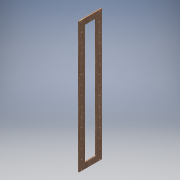
# Autodesk Inventor part: Arm
Saved by Autodesk Inventor 2019 (Build 230136000, 136)
## iProperties
Created: 2019-01-14
Part Number: Arm
Material: Wood (Birch)
Document SubType Name: Modeling
Designer: nxgam
Density: 0.55 g/cm^3
Appearance: Birch - Natural Polished
Author: nxgam
Autodesk Inventor part; units mm, degrees
ref_plane "YZ Plane" through (0, 0, 0) normal (1, 0, 0) x (0, 1, 0)
ref_plane "XZ Plane" through (0, 0, 0) normal (0, 1, 0) x (-1, 0, 0)
ref_plane "XY Plane" through (0, 0, 0) normal (0, 0, 1) x (1, 0, 0)
sketch "Sketch1" plane through (0, 0, 0) normal (1, 0, 0) x (0, 1, 0)
  line L0 (0, 50.8) -> (579.12, 50.8)
  line L1 (579.12, 50.8) -> (579.12, -50.8)
  line L2 (579.12, -50.8) -> (0, -50.8)
  line L3 (0, -50.8) -> (0, 50.8)
  point P0 (0, 0)
  point P1 (0, 0)
  dimension "d0" = 579.12
  dimension "d1" = 101.6
  constraints: 8 end point, 2 parallel, 1 coincident, 1 horizontal, 1 midpoint, 1 perpendicular, 1 other
  measures "d0" distance of L1.end L2.end
  measures "d1" distance of L0.end L1.end
extrude "Extrusion1" add sketch "Sketch1" along normal blind 5.08
sketch "Sketch2" plane through (5.08, 0, 0) normal (1, 0, 0) x (0, 0, -1)
  line L0 (-50.8, 579.12) -> (-50.8, 0) projected
  line L1 (-50.8, 0) -> (50.8, 0) projected
  line L2 (50.8, 0) -> (50.8, 579.12) projected
  line L3 (50.8, 579.12) -> (-50.8, 579.12) projected
  line L4 (-25.4, 553.72) -> (-25.4, 25.4)
  line L5 (-25.4, 25.4) -> (25.4, 25.4)
  line L6 (25.4, 25.4) -> (25.4, 553.72)
  line L7 (25.4, 553.72) -> (-25.4, 553.72)
  point P0 (0, 0)
  dimension "d4" = 50.8
  constraints: 8 end point, 3 other
  measures "d4" distance between parallel lines of L4 L6
extrude "Extrusion2" cut sketch "Sketch2" against normal blind 5.08 contours L7 L6 L5 L4
sketch "Sketch3" plane through (5.08, 0, 0) normal (1, 0, 0) x (0, 0, -1)
  circle A0 centre (-40.64, 45.72) radius 2 projected
  circle A1 centre (40.64, 5.08) radius 2 projected
  circle A2 centre (-40.64, 5.08) radius 2 projected
  circle A3 centre (40.64, 45.72) radius 2 projected
  line L0 (-42.545, 0) -> (42.545, 0) projected
  line L1 (45.72, 3.175) -> (45.72, 62.865) projected
  line L2 (42.545, 66.04) -> (38.735, 66.04) projected
  line L3 (35.56, 62.865) -> (35.56, 10.16) projected
  line L4 (35.56, 10.16) -> (-35.56, 10.16) projected
  line L5 (-35.56, 10.16) -> (-35.56, 62.865) projected
  line L6 (-38.735, 66.04) -> (-42.545, 66.04) projected
  line L7 (-45.72, 62.865) -> (-45.72, 3.175) projected
  arc A4 (-45.72, 3.175) -> (-42.545, 0) centre (-42.545, 3.175) ccw projected
  arc A5 (42.545, 0) -> (45.72, 3.175) centre (42.545, 3.175) ccw projected
  arc A6 (45.72, 62.865) -> (42.545, 66.04) centre (42.545, 62.865) ccw projected
  arc A7 (38.735, 66.04) -> (35.56, 62.865) centre (38.735, 62.865) ccw projected
  arc A8 (-35.56, 62.865) -> (-38.735, 66.04) centre (-38.735, 62.865) ccw projected
  arc A9 (-42.545, 66.04) -> (-45.72, 62.865) centre (-42.545, 62.865) ccw projected
  point P0 (0, 0)
  point P1 (-40.64, 45.72)
  point P2 (40.64, 5.08)
  point P3 (40.64, 45.72)
  point P4 (-40.64, 86.36)
  point P5 (40.64, 86.36)
  point P6 (-40.64, 127)
  point P7 (40.64, 127)
  point P8 (-40.64, 167.64)
  point P9 (40.64, 167.64)
  point P10 (-40.64, 208.28)
  point P11 (40.64, 208.28)
  point P12 (-40.64, 248.92)
  point P13 (40.64, 248.92)
  point P14 (-40.64, 289.56)
  point P15 (40.64, 289.56)
  point P16 (-40.64, 330.2)
  point P17 (40.64, 330.2)
  point P18 (-40.64, 370.84)
  point P19 (40.64, 370.84)
  point P20 (-40.64, 411.48)
  point P21 (40.64, 411.48)
  point P22 (-40.64, 452.12)
  point P23 (40.64, 452.12)
  point P24 (-40.64, 492.76)
  point P25 (40.64, 492.76)
  point P26 (-40.64, 533.4)
  point P27 (40.64, 533.4)
  point P28 (-40.64, 574.04)
  point P29 (40.64, 574.04)
  dimension "d9" = 40.64
  constraints: 4 coincident, 1 vertical, 26 other
  measures "d9" distance of point (-40.64, 45.72) point (-40.64, 86.36)
hole "Hole1" at (5.08, 5.08, 40.64) at (5.08, 45.72, 40.64) at (5.08, 5.08, -40.64) at (5.08, 45.72, -40.64) at (5.08, 86.36, 40.64) at (5.08, 86.36, -40.64) at (5.08, 127, 40.64) at (5.08, 127, -40.64) at (5.08, 167.64, 40.64) at (5.08, 167.64, -40.64) at (5.08, 208.28, 40.64) at (5.08, 208.28, -40.64) at (5.08, 248.92, 40.64) at (5.08, 248.92, -40.64) at (5.08, 289.56, 40.64) at (5.08, 289.56, -40.64) at (5.08, 330.2, 40.64) at (5.08, 330.2, -40.64) at (5.08, 370.84, 40.64) at (5.08, 370.84, -40.64) at (5.08, 411.48, 40.64) at (5.08, 411.48, -40.64) at (5.08, 452.12, 40.64) at (5.08, 452.12, -40.64) at (5.08, 492.76, 40.64) at (5.08, 492.76, -40.64) at (5.08, 533.4, 40.64) at (5.08, 533.4, -40.64) at (5.08, 574.04, 40.64) at (5.08, 574.04, -40.64) direction (-1, 0, 0) diameter 4 end through all
body "Solid1"
